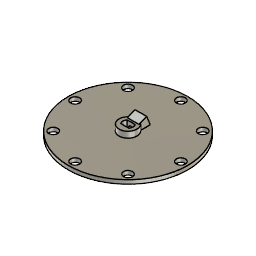
Wheel (Autodesk Fusion 360 design; units mm, degrees)
Autodesk Fusion 360 part; units mm, degrees
sketch "Sketch1" plane through (0, 0, 0) normal (0, 0, 1) x (1, 0, 0)
  circle A0 centre (0, 0) radius 30
  line L0 (0, 0) -> (0, 30) construction
  circle A1 centre (0, 26.55) radius 2.25
  circle A2 centre (-18.7737, 18.7737) radius 2.25
  circle A3 centre (-26.55, 0) radius 2.25
  circle A4 centre (-18.7737, -18.7737) radius 2.25
  circle A5 centre (0, -26.55) radius 2.25
  circle A6 centre (18.7737, -18.7737) radius 2.25
  circle A7 centre (26.55, 0) radius 2.25
  circle A8 centre (18.7737, 18.7737) radius 2.25
  line L1 (-2.0456, 1.564) -> (2.0456, 1.564)
  line L2 (2.0287, -1.5859) -> (-2.0287, -1.5859)
  arc A9 (-2.0456, 1.564) -> (-2.0287, -1.5859) centre (0, 0) ccw
  arc A10 (2.0287, -1.5859) -> (2.0456, 1.564) centre (0, 0) ccw
  circle A11 centre (0, 0) radius 4.5
  dimension "d1" = 60
  dimension "d2" = 4.5
  dimension "d3" = 1.2
  dimension "d5" = 360
  dimension "d6" = 5.15
  dimension "d7" = 3.15
  dimension "d8" = 9
  constraint coincident A0.centre L0.start
  constraint coincident A0 L0.end
  constraint vertical L0
  constraint coincident L0 A1.centre
  constraint horizontal L1
  constraint horizontal L2
  constraint coincident L2.start A9
  constraint concentric A9 A10
  constraint concentric A10 A11
  measures "d1" diameter of A0
  measures "d2" diameter of A1
  measures "d3" distance of L0.end A1
  measures "d6" diameter of A9
  measures "d7" distance of L1.end L2.start
  measures "d8" diameter of A11
extrude "Extrude1" add sketch "Sketch1" along normal blind 2 contours A0 | A11 makes body 1
extrude "Extrude2" add sketch "Sketch1" along normal blind 3 from surface at 2 contours A11 bodies 1
cylinder "CylinderPrimitive1" add diameter 3 height 4.178 placed x (1, 0, 0) y (0, 1, 0) z (0, 0, 1) at (0, 0, 0) separate body makes body 2
move_face "MoveFace1" to x (1, 0, 0) y (0, -1, 0) z (0, 0, -1) at (0, 0, 8.356) 1 faces at (1.4925, -0.1494, 2.7853) on bodies 2
move_body "Move1" bodies 2 to x (1, 0, 0) y (0, 0.368656, -0.929566) z (0, 0.929566, 0.368656) at (0, 0.2997, 1.489)
sketch "Sketch6" plane through (0, 7.8265, 3.1039) normal (0, 0.929566, 0.368656) x (-1, 0, 0)
  line L0 (2.9197, -1.1503) -> (-2.9197, -1.1503)
  line L1 (-2.9197, -1.1503) -> (-2.9197, 3.6976)
  line L2 (-2.9197, 3.6976) -> (2.9197, 3.6976)
  line L3 (2.9197, 3.6976) -> (2.9197, -1.1503)
  circle A0 centre (0, 0.9049) radius 1.5
  line L4 (0, 0.9049) -> (1.5, 0.9049) construction
  line L5 (0, 0.9049) -> (1.0607, 1.9656) construction
  arc A1 (0.8698, 2.127) -> (1.2221, 1.7747) centre (1.0607, 1.9656) ccw
  arc A2 (-1.2221, 1.7747) -> (-0.8698, 2.127) centre (-1.0607, 1.9656) ccw
  arc A3 (-0.8698, -0.3172) -> (-1.2221, 0.0351) centre (-1.0607, -0.1557) ccw
  arc A4 (1.2221, 0.0351) -> (0.8698, -0.3172) centre (1.0607, -0.1557) ccw
  point P0 (0, 1.2737)
  dimension "d56" = 3
  dimension "d67" = 45
  dimension "d68" = 0.5
  dimension "d70" = 360
  constraint horizontal L0
  constraint perpendicular L0 L1
  constraint parallel L0 L2
  constraint parallel L1 L3
  constraint coincident A0.centre L4.start
  constraint coincident A0 L4.end
  constraint perpendicular L3 L4
  constraint coincident A0 L5.end
  constraint coincident L5.end A1.centre
  constraint coincident A0 A1.end
  constraint coincident A0 A1.start
  measures "d56" diameter of A0
  measures "d67" angle of L4 L5
  measures "d68" diameter of A1
extrude "Extrude9" add sketch "Sketch6" against normal blind 4.708 contours L0 L1 L2 L3 | A0 A1 A2 A3 A4 | A0 A1 | A0 A4 | A0 A2 | A0 A3 bodies 1
extrude "Extrude11" cut sketch "Sketch6" against normal blind 7.4022 contours A0 A1 A2 A3 A4 bodies 1
hidden bodies 2
